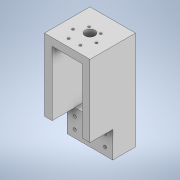
# Autodesk Inventor part: Base_V2c
Saved by Autodesk Inventor 2022 (Build 260153000, 153)
## iProperties
Created: 2022-06-15
Part Number: Base_V2c
Material: Generic
Document SubType Name: Modeling
Designer: Asus
Density: 1 g/cm^3
Appearance: Default
Author: Asus
Autodesk Inventor part; units mm, degrees
ref_plane "YZ Plane" through (0, 0, 0) normal (1, 0, 0) x (0, 1, 0)
ref_plane "XZ Plane" through (0, 0, 0) normal (0, 1, 0) x (-1, 0, 0)
ref_plane "XY Plane" through (0, 0, 0) normal (0, 0, 1) x (1, 0, 0)
sketch "Sketch1" plane through (0, 0, 0) normal (0, 1, 0) x (-1, 0, 0)
  line L0 (30, 30) -> (-30, 30)
  line L1 (-30, 30) -> (-30, -30)
  line L2 (-30, -30) -> (30, -30)
  line L3 (30, -30) -> (30, 30)
  circle A0 centre (0, 0) radius 2.0484
  dimension "d0" = 60
  dimension "d1" = 60
  dimension "d2" = 30
  dimension "d3" = 30
  constraints: 8 end point, 2 parallel, 1 centre point, 1 coincident, 1 horizontal, 1 perpendicular
  measures "d0" distance of L1.end L2.end
  measures "d1" distance of L2.end L0.start
  measures "d2" distance from line of point (0, 0) L3
  measures "d3" distance from line of L0 point (0, 0)
extrude "Extrusion1" add sketch "Sketch1" against normal blind 10
sketch "Sketch2" plane through (0, -10, 0) normal (0, -1, 0) x (1, 0, 0)
  line L0 (30, -30) -> (30, 30) projected
  line L1 (-30, 30) -> (-30, -30) projected
  line L2 (30, 30) -> (-30, 30)
  line L3 (-30, 30) -> (-30, -30)
  line L4 (-30, -30) -> (30, -30)
  line L5 (30, -30) -> (30, 30)
  line L6 (20, 20) -> (-20, 20)
  line L7 (-20, 20) -> (-20, -20)
  line L8 (-20, -20) -> (20, -20)
  line L9 (20, -20) -> (20, 20)
  point P0 (0, 0)
  dimension "d6" = 10
  dimension "d7" = 10
  dimension "d8" = 10
  dimension "d9" = 10
  constraints: 16 end point, 4 parallel, 2 horizontal, 2 perpendicular
  measures "d6" distance between parallel lines of L0 L9
  measures "d7" distance between parallel lines of L2 L6
  measures "d8" distance between parallel lines of L3 L7
  measures "d9" distance between parallel lines of L4 L8
extrude "Extrusion2" add sketch "Sketch2" along normal blind 120
sketch "Sketch3" plane through (-30, 0, 30) normal (0, 0, 1) x (1, 0, 0)
  point P0 (30, 0)
sketch "Sketch4" plane through (-30, 0, 30) normal (0, 0, 1) x (1, 0, 0)
  line L0 (50, -10) -> (10, -10) projected
  line L1 (50, -10) -> (50, -130) projected
  line L2 (10, -10) -> (50, -10)
  line L3 (50, -10) -> (50, -95)
  line L4 (50, -95) -> (10, -95)
  line L5 (10, -95) -> (10, -10)
  point P0 (30, 0)
  dimension "d12" = 85
  constraints: 8 end point, 2 parallel, 1 horizontal, 1 perpendicular, 1 point on line
  measures "d12" distance between parallel lines of L0 L4
extrude "Extrusion3" cut sketch "Sketch4" against normal blind 10
sketch "Sketch5" plane through (-30, 0, 30) normal (0, 0, 1) x (1, 0, 0)
  line L0 (60, 0) -> (60, -130) projected
  line L1 (60, -130) -> (0, -130) projected
  line L2 (60, -95) -> (0, -95)
  line L3 (0, -95) -> (0, -130)
  line L4 (0, -130) -> (60, -130)
  line L5 (60, -130) -> (60, -95)
  point P0 (30, 0)
  dimension "d16" = 35
  constraints: 8 end point, 2 parallel, 1 horizontal, 1 perpendicular, 1 point on line
  measures "d16" distance between parallel lines of L1 L2
extrude "Extrusion4" cut sketch "Sketch5" against normal blind 30
sketch "Sketch6" plane through (-20, -10, -20) normal (0, 0, 1) x (1, 0, 0)
  line L0 (-10, -85) -> (0, -85) projected
  line L1 (0, -85) -> (40, -85)
  line L2 (40, -85) -> (40, -120)
  line L3 (40, -120) -> (0, -120)
  line L4 (0, -120) -> (0, -85)
  point P0 (20, 10)
  constraints: 8 end point, 2 parallel, 1 horizontal, 1 perpendicular
extrude "Extrusion5" add sketch "Sketch6" along normal blind 20
sketch "Sketch7" plane through (-30, 0, 0) normal (0, 0, 1) x (1, 0, 0)
  circle A0 centre (10, -105) radius 1.95
  circle A1 centre (10, -120) radius 1.95
  circle A2 centre (50, -105) radius 1.95
  circle A3 centre (50, -120) radius 1.95
  line L0 (60, -95) -> (60, -130) projected
  line L1 (60, -130) -> (0, -130) projected
  line L2 (50, -95) -> (60, -95) projected
  line L3 (50, -95) -> (10, -95) projected
  line L4 (0, -130) -> (0, -95) projected
  point P0 (30, 0)
  dimension "d21" = 10
  dimension "d22" = 10
  dimension "d23" = 10
  dimension "d24" = 10
  dimension "d25" = 10
  dimension "d26" = 10
  dimension "d27" = 10
  dimension "d28" = 10
  dimension "d29" = 3.9
  dimension "d30" = 3.9
  dimension "d31" = 3.9
  dimension "d32" = 3.9
  constraints: 4 centre point
  measures "d21" distance from line of L0 A3.centre
  measures "d22" distance from line of L1 A3.centre
  measures "d23" distance from line of L2 A2.centre
  measures "d24" distance from line of L0 A2.centre
  measures "d25" distance from line of L3 A0.centre
  measures "d26" distance from line of L4 A0.centre
  measures "d27" distance from line of L4 A1.centre
  measures "d28" distance from line of L1 A1.centre
  measures "d29" diameter of A1
  measures "d30" diameter of A0
  measures "d31" diameter of A2
  measures "d32" diameter of A3
extrude "Extrusion6" cut sketch "Sketch7" against normal blind 35
sketch "Sketch8" plane through (30, 0, -30) normal (0, 0, -1) x (-1, 0, 0)
  circle A0 centre (10, -105) radius 1.95 projected
  circle A1 centre (10, -105) radius 4.5
  circle A2 centre (10, -120) radius 1.95 projected
  circle A3 centre (10, -120) radius 4.5
  circle A4 centre (50, -105) radius 1.95 projected
  circle A5 centre (50, -105) radius 4.5
  circle A6 centre (50, -120) radius 1.95 projected
  circle A7 centre (50, -120) radius 4.5
  point P0 (30, 0)
  dimension "d35" = 9
  dimension "d36" = 9
  dimension "d37" = 9
  dimension "d38" = 9
  constraints: 4 centre point, 4 coincident
  measures "d35" diameter of A1
  measures "d36" diameter of A5
  measures "d37" diameter of A7
  measures "d38" diameter of A3
extrude "Extrusion7" cut sketch "Sketch8" against normal blind 15 contours A0 | A1 | A3 | A5 | A7
sketch "Sketch9" plane through (0, 0, 0) normal (0, 1, 0) x (1, 0, 0)
  circle A0 centre (0, 0) radius 6.5
  circle A1 centre (0, -7) radius 15.5
  line L0 (30, -30) -> (30, 30) projected
  line L1 (0, -7) -> (-17.1994, -7)
  line L2 (-17.1994, -7) -> (16.6076, -7)
  line L3 (0, -7) -> (-8.5199, -21.7569)
  line L4 (0, -7) -> (9.3939, -23.2707)
  line L5 (0, -7) -> (10.7829, 11.6765)
  line L6 (0, -7) -> (-10.6515, 11.4489)
  circle A2 centre (7.75, 6.4234) radius 1.5
  circle A3 centre (-7.75, 6.4234) radius 1.5
  circle A4 centre (-15.5, -7) radius 1.5
  circle A5 centre (-7.75, -20.4234) radius 1.5
  circle A6 centre (7.75, -20.4234) radius 1.5
  circle A7 centre (15.5, -7) radius 1.5
  dimension "d44" = 13
  dimension "d45" = 31
  dimension "d46" = 7
  dimension "d47" = 30
  dimension "d48" = 60
  dimension "d49" = 60
  dimension "d50" = 60
  dimension "d51" = 60
  dimension "d52" = 3
  dimension "d53" = 3
  dimension "d54" = 3
  dimension "d55" = 3
  dimension "d56" = 3
  dimension "d57" = 3
  constraints: 12 end point, 8 centre point, 7 point on line, 6 point on circle, 1 coincident, 1 horizontal
  measures "d44" diameter of A0
  measures "d45" diameter of A1
  measures "d46" distance of L1.start point (0, 0)
  measures "d47" distance from line of L0 L1.start
  measures "d48" angle of L3 L1
  measures "d49" angle of L4 L3
  measures "d50" angle of L5 L2
  measures "d51" angle of L1 L6
  measures "d52" diameter of A7
  measures "d53" diameter of A4
  measures "d54" diameter of A3
  measures "d55" diameter of A2
  measures "d56" diameter of A6
  measures "d57" diameter of A5
extrude "Extrusion8" cut sketch "Sketch9" against normal blind 10 contours A0 L5 | L5 A0 L6 | L6 A0 | A2 A1 L5 | L5 A1 A2 | A3 A1 L6 | L6 A1 A3 | L5 A2 A1 | A1 A2 L5 | A4 A1 L1 | L1 A1 A4 | A7 A1 L2 | L2 A1 A7 | A5 A1 L3 | L3 A1 A5 | A6 A1 L4 | L4 A1 A6 | L6 A3 A1 | A1 A3 L6 | A7 A1 | L1 A4 A1 | A1 A4 L1 | L3 A5 A1 | A1 A5 L3 | L4 A6 A1 | A1 A6 L4 picked at (0.3591, 1.0442)
body "Solid1"
